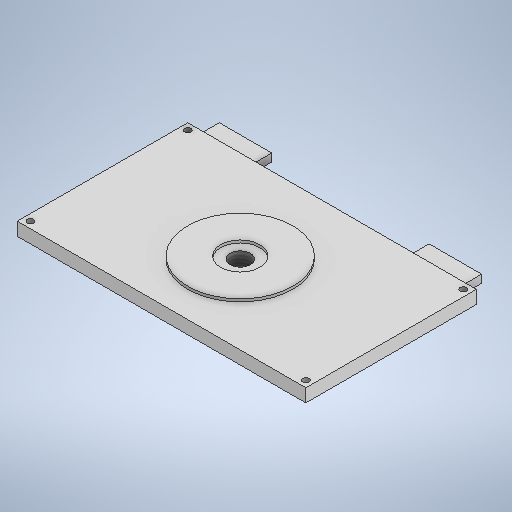
# Autodesk Inventor part: chassis_haut
Saved by Autodesk Inventor 2026.2 (Build 302298010, 298A)
## iProperties
Created: 2026-03-16
Part Number: chassis_haut
Material: Générique
Document SubType Name: Modeling
Designer: genon
Density: 1 g/cm^3
Appearance: Par défaut
Author: genon
Autodesk Inventor part; units mm, degrees
ref_plane "YZ Plane" through (0, 0, 0) normal (1, 0, 0) x (0, 1, 0)
ref_plane "XZ Plane" through (0, 0, 0) normal (0, 1, 0) x (-1, 0, 0)
ref_plane "XY Plane" through (0, 0, 0) normal (0, 0, 1) x (1, 0, 0)
sketch "Esquisse1" plane through (0, 0, 0) normal (0, 1, 0) x (-1, 0, 0)
  line L0 (-55, 100) -> (55, 100)
  line L1 (55, 100) -> (55, -100)
  line L2 (55, -100) -> (-55, -100)
  line L3 (-55, -100) -> (-55, 100)
  line L4 (-55, 100) -> (55, -100) construction
  line L5 (55, 100) -> (-55, -100) construction
  point P0 (0, 0)
  dimension "d0" = 110
  dimension "d1" = 200
  constraints: 12 end point, 2 midpoint, 2 parallel, 1 horizontal, 1 perpendicular
  measures "d0" distance of L1.end L2.end
  measures "d1" distance of L0.end L1.end
extrude "Extrusion1" add sketch "Esquisse1" along normal blind 5
sketch "Esquisse4" plane through (0, 5, 0) normal (0, 1, 0) x (1, 0, 0)
  line L0 (0, 0) -> (0, 60)
  dimension "d22" = 60
  constraints: 2 end point, 1 coincident, 1 vertical
  measures "d22" distance of L0.start L0.end
hole "Perçage3" at (0, 5, -60) direction (0, -1, 0) diameter 7.6468 end through all thread size "M9x1.25" class "6H" standard "ISO Metric profile"
sketch "Esquisse5" plane through (0, 5, 0) normal (0, 1, 0) x (1, 0, 0)
  line L0 (-55, -100) -> (55, -100) projected
  line L1 (0, -100) -> (-27.5, -100)
  line L2 (-27.5, -100) -> (-27.5, -70)
  line L3 (-27.5, -70) -> (-37.5, -70)
  line L4 (-27.5, -70) -> (-7.5, -70)
  line L5 (-37.5, -70) -> (-37.5, -55)
  line L6 (-7.5, -55) -> (-7.5, -70)
  point P0 (0, 0)
  dimension "d30" = 27.5
  dimension "d31" = 30
  dimension "d32" = 10
  dimension "d33" = 20
  dimension "d34" = 15
  constraints: 12 end point, 4 coincident, 2 horizontal, 2 vertical, 1 midpoint, 1 perpendicular, 1 point on line
  measures "d30" distance of L1.start L1.end
  measures "d31" distance of L1.end L2.end
  measures "d32" distance of L2.end L3.end
  measures "d33" distance of L2.end L4.end
  measures "d34" distance of L5.start L5.end
hole "Perçage4" at (-7.5, 5, 70) at (-37.5, 5, 70) at (-37.5, 5, 55) at (-7.5, 5, 55) direction (0, -1, 0) diameter 2.459 end through all thread size "M3x0.5" class "6H" standard "ISO Metric profile"
sketch "Esquisse6" plane through (-55, 0, 100) normal (0, 0, 1) x (1, 0, 0)
  line L0 (0, 0) -> (110, 0) projected
  line L1 (110, 0) -> (110, 5) projected
  line L2 (0, 5) -> (110, 5) projected
  line L3 (0, 0) -> (0, 5) projected
  point P0 (55, 0)
extrude "Extrusion2" add sketch "Esquisse6" along normal blind 40
sketch "Esquisse7" plane through (0, 5, 0) normal (0, 1, 0) x (1, 0, 0)
  circle A0 centre (0, 60) radius 3.8234 projected
  circle A1 centre (0, 60) radius 7.5
  circle A2 centre (0, 60) radius 20
  point P0 (0, 0)
  dimension "d47" = 15
  dimension "d48" = 40
  constraints: 2 centre point, 2 coincident
  measures "d47" diameter of A1
  measures "d48" diameter of A2
extrude "Extrusion3" add sketch "Esquisse7" along normal blind 1 contours A2
sketch "Esquisse8" plane through (0, 5, 0) normal (0, 1, 0) x (1, 0, 0)
  line L0 (-55, 100) -> (-55, -140) projected
  line L1 (55, 100) -> (55, -140) projected
  line L2 (-55, -140) -> (55, -140)
  line L3 (55, -140) -> (55, 30)
  line L4 (55, 30) -> (-55, 30)
  line L5 (-55, 30) -> (-55, -140)
  point P0 (0, 0)
  dimension "d51" = 170
  constraints: 8 end point, 2 parallel, 1 horizontal, 1 perpendicular, 1 point on line
  measures "d51" distance of L3.end L2.end
extrude "Extrusion4" cut sketch "Esquisse8" against normal blind 10
sketch "Esquisse9" plane through (0, 5, 0) normal (0, 1, 0) x (1, 0, 0)
  line L0 (-55, 30) -> (55, 30) projected
  line L1 (-55, 30) -> (-55, 32.5)
  line L2 (-55, 100) -> (-55, 30) projected
  line L3 (-55, 32.5) -> (-52.5, 32.5)
  line L4 (55, 30) -> (55, 32.5)
  line L5 (55, 100) -> (55, 30) projected
  line L6 (55, 32.5) -> (52.5, 32.5)
  point P0 (0, 0)
  dimension "d54" = 2.5
  dimension "d55" = 2.5
  dimension "d56" = 2.5
  dimension "d57" = 2.5
  constraints: 8 end point, 2 coincident, 2 perpendicular, 2 point on line
  measures "d54" distance of L0.start L1.end
  measures "d55" distance of L1.end L3.end
  measures "d56" distance of L0.end L4.end
  measures "d57" distance of L4.end L6.end
hole "Perçage5" at (-52.5, 5, -32.5) at (52.5, 5, -32.5) direction (0, -1, 0) diameter 2.459 end through all thread size "M3x0.5" class "6H" standard "ISO Metric profile"
sketch "Esquisse10" plane through (0, 5, 0) normal (0, 1, 0) x (1, 0, 0)
  line L0 (55, 100) -> (-55, 100) projected
  line L1 (55, 100) -> (55, 30) projected
  line L2 (-55, 100) -> (55, 100)
  line L3 (55, 100) -> (55, 95)
  line L4 (55, 95) -> (-55, 95)
  line L5 (-55, 95) -> (-55, 100)
  point P0 (0, 0)
  dimension "d65" = 5
  constraints: 8 end point, 2 parallel, 1 horizontal, 1 perpendicular, 1 point on line
  measures "d65" distance of L2.end L3.end
extrude "Extrusion5" cut sketch "Esquisse10" against normal blind 10
sketch "Esquisse11" plane through (0, 5, 0) normal (0, 1, 0) x (1, 0, 0)
  line L0 (-55, 95) -> (-52.5, 95)
  line L1 (55, 95) -> (-55, 95) projected
  line L2 (-52.5, 95) -> (-52.5, 92.5)
  line L3 (55, 95) -> (55, 30) projected
  line L4 (55, 95) -> (52.5, 95)
  line L5 (52.5, 95) -> (52.5, 92.5)
  point P0 (0, 0)
  dimension "d68" = 2.5
  dimension "d69" = 2.5
  dimension "d70" = 2.5
  constraints: 8 end point, 2 coincident, 2 perpendicular, 2 point on line
  measures "d68" distance of L0.start L0.end
  measures "d69" distance of L0.end L2.end
  measures "d70" distance of L1.start L4.end
hole "Perçage6" at (-52.5, 5, -92.5) at (52.5, 5, -92.5) direction (0, -1, 0) diameter 2.459 end through all thread size "M3x0.5" class "6H" standard "ISO Metric profile"
sketch "Esquisse12" plane through (55, 5, -95) normal (0, 0, -1) x (-1, 0, 0)
  line L0 (0, -5) -> (0, 0) projected
  line L1 (0, 0) -> (5, 0)
  line L2 (110, 0) -> (0, 0) projected
  line L3 (5, 0) -> (5, -1)
  line L4 (5, -1) -> (25, -1)
  line L5 (25, -1) -> (25, -4)
  line L6 (25, -4) -> (5, -4)
  line L7 (5, -4) -> (5, -1)
  line L8 (110, -5) -> (110, 0) projected
  line L9 (110, 0) -> (105, 0)
  line L10 (105, 0) -> (105, -1)
  line L11 (105, -1) -> (85, -1)
  line L12 (85, -1) -> (85, -4)
  line L13 (85, -4) -> (105, -4)
  line L14 (105, -4) -> (105, -1)
  point P0 (55, -5)
  dimension "d78" = 5
  dimension "d79" = 1
  dimension "d80" = 20
  dimension "d81" = 3
  dimension "d82" = 5
  dimension "d83" = 20
  constraints: 24 end point, 4 parallel, 4 perpendicular, 2 horizontal, 2 point on line
  measures "d78" distance of L0.end L1.end
  measures "d79" distance of L1.end L3.end
  measures "d80" distance of L5.end L6.end
  measures "d81" distance of L4.end L5.end
  measures "d82" distance of L2.start L9.end
  measures "d83" distance of L13.end L12.end
extrude "Extrusion6" add sketch "Esquisse12" along normal blind 7
